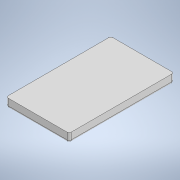
# Autodesk Inventor part: Monitor
Saved by Autodesk Inventor 2020 (Build 240168000, 168)
## iProperties
Created: 2019-11-09
Part Number: Monitor
Material: Generic
Document SubType Name: Modeling
Designer: nicoc
Density: 1 g/cm^3
Appearance: Default
Author: nicoc
Autodesk Inventor part; units mm, degrees
ref_plane "YZ Plane" through (0, 0, 0) normal (1, 0, 0) x (0, 1, 0)
ref_plane "XZ Plane" through (0, 0, 0) normal (0, 1, 0) x (-1, 0, 0)
ref_plane "XY Plane" through (0, 0, 0) normal (0, 0, 1) x (1, 0, 0)
sketch "Sketch1" plane through (0, 0, 0) normal (0, 1, 0) x (-1, 0, 0)
  line L0 (0, 0) -> (293.4, 0)
  line L1 (293.4, 0) -> (293.4, -487.3)
  line L2 (293.4, -487.3) -> (0, -487.3)
  line L3 (0, -487.3) -> (0, 0)
  dimension "d0" = 293.4
  dimension "d1" = 487.3
  constraints: 8 end point, 2 parallel, 1 horizontal, 1 perpendicular
  measures "d0" distance between parallel lines of L1 L3
  measures "d1" distance between parallel lines of L2 L0
extrude "Extrusion1" add sketch "Sketch1" along normal blind 41.3
fillet "Fillet1" radius 10 4 edges at (0, 0, -243.65) (-146.7, 0, 0) (-293.4, 0, -243.65) (-146.7, 0, -487.3)
fillet "Fillet2" radius 10 8 edges at (-2.9289, 2.9289, -484.3711) (0, 25.65, -487.3) (-290.4711, 2.9289, -484.3711) (-293.4, 25.65, -487.3) (-2.9289, 2.9289, -2.9289) (0, 25.65, 0) (-293.4, 25.65, 0) (-290.4711, 2.9289, -2.9289)
sketch "Sketch2" plane through (0, 0, 0) normal (0, -1, 0) x (1, 0, 0)
  line L0 (-283.4, -487.3) -> (-10, -487.3) projected
  line L1 (-293.4, -10) -> (-293.4, -477.3) projected
  point P0 (0, 0)
  point P1 (-196.7, -293.65)
  point P2 (-196.7, -193.65)
  point P3 (-96.7, -293.65)
  point P4 (-96.7, -193.65)
  dimension "d6" = 193.65
  dimension "d8" = 96.7
  dimension "d9" = 100
  dimension "d10" = 96.7
  dimension "d11" = 193.65
  dimension "d12" = 100
  dimension "d13" = 100
  dimension "d14" = 100
  measures "d6" distance from line of L0 point (-196.7, -293.65)
  measures "d8" distance from line of L1 point (-196.7, -293.65)
  measures "d9" distance of point (-196.7, -193.65) point (-196.7, -293.65)
  measures "d10" distance from line of L1 point (-196.7, -193.65)
  measures "d11" distance from line of L0 point (-96.7, -293.65)
  measures "d12" distance of point (-96.7, -193.65) point (-96.7, -293.65)
  measures "d13" distance of point (-96.7, -293.65) point (-196.7, -293.65)
  measures "d14" distance of point (-96.7, -193.65) point (-196.7, -193.65)
hole "Hole1" at (-196.7, 0, -293.65) at (-196.7, 0, -193.65) at (-96.7, 0, -293.65) at (-96.7, 0, -193.65) direction (0, 1, 0) diameter 4.5 depth 5
equation "\"d10\" = d8"
equation "\"d11\" = d6"
equation "\"d12\" = d9"
equation "\"d13\" = d9"
equation "\"d14\" = d9"
body "Solid1"
